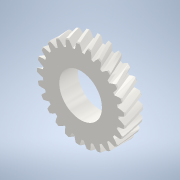
# Autodesk Inventor part: Цилиндрическое зубчатое зацепление1
Saved by Autodesk Inventor 2021 (Build 250183000, 183)
## iProperties
CustomPartVersion: 1
Created: 2021-03-22
Part Number: Цилиндрическое зубчатое зацепление1
Material: Steel
Document SubType Name: Modeling
Designer: Данил
Categories: <?xml version="1.0" encoding="UTF-16"?> <MemberInstance><Categories><FamilyTemplate><FamilyTemplateParameter ValueType="xs:double" Id="1" ObjectReferenceKey="da_z" ObjectType="kUserParameterObject"/><FamilyTemplateParameter ValueType="xs:double" Id="2" ObjectReferenceKey="da_b" ObjectType="kUserParameterObject"/><FamilyTemplateParameter ValueType="xs:double" Id="3" ObjectReferenceKey="da_beta" ObjectType="kUserParameterObject"/><FamilyTemplateParameter ValueType="xs:double" Id="4" ObjectReferenceKey="da_da" ObjectType="kUserParameterObject"/><FamilyTemplateParameter ValueType="xs:double" Id="5" ObjectReferenceKey="da_aw" ObjectType="kUserParameterObject"/><FamilyTemplateParameter ValueType="xs:string" Id="6" ObjectReferenceKey="EAIAABAAAACIAQAAAAAAAIAAAAAAAAAA" ObjectType="83910656" SubObjectId="SurfaceGeometry"/></FamilyTemplate><ParamToTemplateMap><ParamToTemplate CategoryParameter="//CategoryParameter[@InternalName='046C89C9-8512-4d59-83FE-43B91F4F132A']" TemplateParameter="1"/><ParamToTemplate CategoryParameter="//CategoryParameter[@InternalName='2552DF32-E462-4b46-AEBF-C6C7768E72AC']" TemplateParameter="2"/><ParamToTemplate CategoryParameter="//CategoryParameter[@InternalName='C9EE641D-15FC-4fae-A226-E94C4372FDD7']" TemplateParameter="3"/><ParamToTemplate><ParamToTemplate CategoryParameter="//CategoryParameter[@InternalName='00B6519A-459B-49c7-AD84-2E56D39A5744']" ConstantValue="0.314300"/></ParamToTemplate><ParamToTemplate><ParamToTemplate CategoryParameter="//CategoryParameter[@InternalName='04B31F0E-C7A6-4894-AA32-9629BEFACF47']" ConstantValue="1.000000"/></ParamToTemplate><ParamToTemplate><ParamToTemplate CategoryParameter="//CategoryParameter[@InternalName='43CBEC2E-7847-49e7-A936-2F7889FCB2D9']" ConstantValue="0.250000"/></ParamToTemplate><ParamToTemplate><ParamToTemplate CategoryParameter="//CategoryParameter[@InternalName='B1EFC894-105D-4ebd-86BF-FA20ED196853']" ConstantValue="0.300000"/></ParamToTemplate><ParamToTemplate><ParamToTemplate CategoryParameter="//CategoryParameter[@InternalName='51175063-3D10-4879-93E8-6246FE8B403D']" ConstantValue="2060000000.000000"/></ParamToTemplate><ParamToTemplate><ParamToTemplate CategoryParameter="//CategoryParameter[@InternalName='A3A52E27-4454-46a9-B0BD-C932399B70AF']" ConstantValue="0.300000"/></ParamToTemplate><ParamToTemplate><ParamToTemplate CategoryParameter="//CategoryParameter[@InternalName='91B76062-C214-41d9-B1B9-14D2AB99603D']" ConstantValue="0.350000"/></ParamToTemplate><ParamToTemplate><ParamToTemplate CategoryParameter="//CategoryParameter[@InternalName='374E806E-8B8A-4dda-A9AA-1039D6500AD2']" ConstantValue="2.857143"/></ParamToTemplate><ParamToTemplate><ParamToTemplate CategoryParameter="//CategoryParameter[@InternalName='2D373A89-B862-43d6-8D0B-0CBF12AB9F6C']" ConstantValue="0.349066"/></ParamToTemplate><ParamToTemplate CategoryParameter="//CategoryParameter[@InternalName='37777632-D6A2-4fac-9D53-DB8ACD95C989']" TemplateParameter="4"/><ParamToTemplate CategoryParameter="//CategoryParameter[@InternalName='FD1017F1-B727-4f7e-9707-0F86F1FF9423']" TemplateParameter="5"/><ParamToTemplate><ParamToTemplate CategoryParameter="//CategoryParameter[@InternalName='9E1B4470-B2D3-4ff1-B813-535BB4CDF51A']" ConstantValue="3520000.000000"/></ParamToTemplate><ParamToTemplate><ParamToTemplate CategoryParameter="//CategoryParameter[@InternalName='F8452263-BFF6-458c-9FB1-07C4B99E95CD']" ConstantValue="11400000.000000"/></ParamToTemplate><ParamToTemplate><ParamToTemplate CategoryParameter="//CategoryParameter[@InternalName='3E3BB259-FD49-497f-8171-6EBC954A3479']" ConstantValue="2.000000"/></ParamToTemplate><ParamToTemplate CategoryParameter="//CategoryParameter[@InternalName='27C3BAF2-7550-4e4b-AE2C-0DB134B7D9B7']" TemplateParameter="6"/></ParamToTemplateMap><Category DisplayName="Gear" InternalName="DC85795E-93AB-48d5-8EEE-5A27447B64BD" Mnemonic="Gear"><CategoryParameter DisplayName="z" InternalName="046C89C9-8512-4d59-83FE-43B91F4F132A" Mnemonic="z"/><CategoryParameter DisplayName="b" InternalName="2552DF32-E462-4b46-AEBF-C6C7768E72AC" Mnemonic="b"/><CategoryParameter DisplayName="||b|" InternalName="C9EE641D-15FC-4fae-A226-E94C4372FDD7" Mnemonic="beta"/><CategoryParameter DisplayName="x" InternalName="00B6519A-459B-49c7-AD84-2E56D39A5744" Mnemonic="x"/><CategoryParameter DisplayName="a*" InternalName="04B31F0E-C7A6-4894-AA32-9629BEFACF47" Mnemonic="a"/><CategoryParameter DisplayName="c*" InternalName="43CBEC2E-7847-49e7-A936-2F7889FCB2D9" Mnemonic="c"/><CategoryParameter DisplayName="r|.f|*" InternalName="B1EFC894-105D-4ebd-86BF-FA20ED196853" Mnemonic="rf"/><CategoryParameter DisplayName="E" InternalName="51175063-3D10-4879-93E8-6246FE8B403D" Mnemonic="E"/><CategoryParameter DisplayName="||m|" InternalName="A3A52E27-4454-46a9-B0BD-C932399B70AF" Mnemonic="mi"/><Category DisplayName="SpurGear" InternalName="26C5A22E-A91E-4dfd-A3B3-23CCAFAE1764" Mnemonic="SpurGear"><CategoryParameter DisplayName="m" InternalName="91B76062-C214-41d9-B1B9-14D2AB99603D" Mnemonic="m"/><CategoryParameter DisplayName="P" InternalName="374E806E-8B8A-4dda-A9AA-1039D6500AD2" Mnemonic="PP"/><CategoryParameter DisplayName="||a|" InternalName="2D373A89-B862-43d6-8D0B-0CBF12AB9F6C" Mnemonic="alpha"/><CategoryParameter DisplayName="d|.a|" InternalName="37777632-D6A2-4fac-9D53-DB8ACD95C989" Mnemonic="da"/><CategoryParameter DisplayName="a|.w|" InternalName="FD1017F1-B727-4f7e-9707-0F86F1FF9423" Mnemonic="aw"/><CategoryParameter DisplayName="||s||.Flim|" InternalName="9E1B4470-B2D3-4ff1-B813-535BB4CDF51A" Mnemonic="sFlim"/><CategoryParameter DisplayName="||s||.Hlim|" InternalName="F8452263-BFF6-458c-9FB1-07C4B99E95CD" Mnemonic="sHlim"/><CategoryParameter DisplayName="тип" InternalName="3E3BB259-FD49-497f-8171-6EBC954A3479" Mnemonic="type"/><CategoryParameter DisplayName="PitchDiameter" InternalName="27C3BAF2-7550-4e4b-AE2C-0DB134B7D9B7" Mnemonic="IDS_PITCHDIAM"/></Category></Category></Categories></MemberInstance>
Density: 1 g/cm^3
Appearance: Steel
Author: Данил
Autodesk Inventor part; units mm, degrees
ref_plane "YZ Plane" through (0, 0, 0) normal (1, 0, 0) x (0, 1, 0)
ref_plane "XZ Plane" through (0, 0, 0) normal (0, 1, 0) x (-1, 0, 0)
ref_plane "XY Plane" through (0, 0, 0) normal (0, 0, 1) x (1, 0, 0)
sketch "Sketch1" plane through (0, 0, 0) normal (0, 0, 1) x (1, 0, 0)
  circle A0 centre (0, 0) radius 52.1283
  dimension "d0" = 104.2566
  constraints: 1 centre point
  measures "d0" diameter of A0
extrude "Extrusion1" add sketch "Sketch1" along normal blind 22
ref_plane "Work Plane2" through (0, 0, 11) normal (0, 0, 1) x (1, 0, 0)
sketch "Sketch2" plane through (0, 0, 0) normal (0, 0, -1) x (-1, 0, 0)
  circle A0 centre (0, 0) radius 52.1283 projected
  circle A1 centre (0, 0) radius 47.5283
  dimension "d3" = 95.0565
  constraints: 1 centre point, 1 coincident
  measures "d3" diameter of A1
surface extrude "Средний диаметр" sketch "Sketch2" against normal through all shown no curves A1
ref_plane "Work Plane8" through (0, 0, 0) normal (0.9921147, 0.1253332, 0) x (0, 0, 1)
ref_plane "Work Plane9" through (0, 0, 0) normal (1, 0, 0) x (0, 1, 0)
spur gear teeth "Цилиндрическое зубчатое зацепление" teeth 25 pitch diameter 95.0565 tip diameter 104.2566 root diameter 88.5066 face width 22 helix angle 23 hand left start plane through (0, 0, 0) normal (0, 0, -1) x (-1, 0, 0)
sketch "Эскиз3" plane through (0, 0, 22) normal (0, 0, 1) x (1, 0, 0)
  circle A0 centre (0, 0) radius 25
  dimension "d49" = 50
  constraints: 1 centre point, 1 coincident
  measures "d49" diameter of A0
extrude "Выдавливание2" cut sketch "Эскиз3" against normal through all
chamfer "Фаска1" distance 1 angle 45 25 edges at (0, 52.1283, 0) (-12.9638, 50.4906, 0) (-25.113, 45.6804, 0) (-35.6843, 37.9999, 0) (-44.0134, 27.9317, 0) (-49.577, 16.1085, 0) (-52.0255, 3.2732, 0) (-51.205, -9.7679, 0) (-47.1671, -22.1952, 0) (-40.1656, -33.2278, 0) (-30.6403, -42.1727, 0) (-19.1897, -48.4677, 0) (-6.5334, -51.7173, 0) (6.5334, -51.7173, 0) (19.1897, -48.4677, 0) (30.6403, -42.1727, 0) (40.1656, -33.2278, 0) (47.1671, -22.1952, 0) (51.205, -9.7679, 0) (52.0255, 3.2732, 0) (49.577, 16.1085, 0) (44.0134, 27.9317, 0) (35.6843, 37.9999, 0) (25.113, 45.6804, 0) (12.9638, 50.4906, 0) measured on face at (-49.1014, 15.954, 0) measured on face at (-19.0057, -48.0028, 0) measured on face at (30.3464, -41.7682, 0) measured on face at (0, 51.6283, 0) measured on face at (-24.8721, 45.2422, 0) measured on face at (43.5912, 27.6638, 0) measured on face at (19.0057, -48.0028, 0) measured on face at (49.1014, 15.954, 0) measured on face at (46.7147, -21.9823, 0) measured on face at (-43.5912, 27.6638, 0) measured on face at (50.7138, -9.6742, 0) measured on face at (-39.7803, -32.9091, 0) measured on face at (35.342, 37.6354, 0) measured on face at (-30.3464, -41.7682, 0) measured on face at (-35.342, 37.6354, 0) measured on face at (12.8394, 50.0063, 0) measured on face at (-46.7147, -21.9823, 0) measured on face at (6.4707, -51.2212, 0) measured on face at (-12.8394, 50.0063, 0) measured on face at (-51.5264, 3.2418, 0) measured on face at (-50.7138, -9.6742, 0) measured on face at (39.7803, -32.9091, 0) measured on face at (51.5264, 3.2418, 0) measured on face at (-6.4707, -51.2212, 0) measured on face at (24.8721, 45.2422, 0)
chamfer "Фаска2" distance 1 angle 45 25 edges at (-2.8576, 52.0499, 22) (10.1765, 51.1253, 22) (22.5711, 46.9883, 22) (33.5476, 39.8989, 22) (42.4161, 30.3025, 22) (48.6194, 18.802, 22) (51.7678, 6.1202, 22) (51.6634, -6.9462, 22) (48.3129, -19.5762, 22) (41.9266, -30.9761, 22) (32.906, -40.4296, 22) (21.8178, -47.3429, 22) (9.3586, -51.2814, 22) (-3.6886, -51.9977, 22) (-16.504, -49.4467, 22) (-28.2824, -43.7889, 22) (-38.2837, -35.3797, 22) (-45.8795, -24.7474, 22) (-50.5925, -12.5601, 22) (-52.1267, 0.4163, 22) (-50.3855, 13.3666, 22) (-45.4784, 25.477, 22) (-37.7137, 35.9866, 22) (-27.5794, 44.2351, 22) (-15.7121, 49.704, 22) measured on face at (-16.3457, -48.9725, 22) measured on face at (48.153, 18.6217, 22) measured on face at (-51.6267, 0.4123, 22) measured on face at (33.2258, 39.5162, 22) measured on face at (-37.352, 35.6415, 22) measured on face at (51.2713, 6.0615, 22) measured on face at (-15.5614, 49.2273, 22) measured on face at (21.6085, -46.8888, 22) measured on face at (-45.0422, 25.2327, 22) measured on face at (47.8495, -19.3884, 22) measured on face at (-37.9165, -35.0403, 22) measured on face at (-49.9022, 13.2384, 22) measured on face at (-3.6532, -51.4989, 22) measured on face at (-28.0111, -43.3689, 22) measured on face at (9.2689, -50.7895, 22) measured on face at (-27.3148, 43.8108, 22) measured on face at (22.3546, 46.5377, 22) measured on face at (-2.8302, 51.5507, 22) measured on face at (10.0789, 50.635, 22) measured on face at (-45.4394, -24.51, 22) measured on face at (51.1679, -6.8796, 22) measured on face at (32.5904, -40.0419, 22) measured on face at (-50.1073, -12.4397, 22) measured on face at (42.0092, 30.0118, 22) measured on face at (41.5245, -30.679, 22)
equation "\"d0\" = da_da"
equation "\"d1\" = da_b"
equation "\"d3\" = da_d"
equation "\"d16\" = da_aw"
equation "\"d43\" = da_aw"
equation "\"d46\" = da_aw"
equation "\"da_da\" = 104.256633"
equation "\"da_b\" = 22"
equation "\"da_d\" = 95.056533"
equation "\"da_aw\" = 184.409674"
body "Solid1"
body "Srf1"
